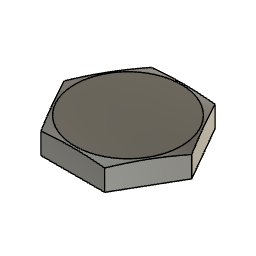
Main Wheel Holder (Autodesk Fusion 360 design; units mm, degrees)
Autodesk Fusion 360 part; units mm, degrees
sketch "Sketch1" plane through (0, 0, 0) normal (0, 0, 1) x (1, 0, 0) in component "Component"
  circle A0 centre (0, 0) radius 1.55
  circle A1 centre (0, 0) radius 2.75
  line L0 (-2.75, 0) -> (-1.375, -2.3816)
  line L1 (-1.375, -2.3816) -> (1.375, -2.3816)
  line L2 (1.375, -2.3816) -> (2.75, 0)
  line L3 (2.75, 0) -> (1.375, 2.3816)
  line L4 (1.375, 2.3816) -> (-1.375, 2.3816)
  line L5 (-1.375, 2.3816) -> (-2.75, 0)
  dimension "d1" = 3.1
  dimension "d2" = 5.5
  dimension "d12" = 4.7631
  constraint coincident A0.centre A1.centre
  constraint concentric A0 A1
  constraint coincident A1 L0.start
  measures "d1" diameter of A0
  measures "d2" diameter of A1
  measures "d12" distance of L0 L3
extrude "Extrude1" add sketch "Sketch1" along normal blind 1 contours A0 | L0 L1 L2 L3 L4 L5 in component "Component"
extrude "Extrude2" cut sketch "Sketch1" along normal blind 0.5 contours A0 in component "Component"
extrude "Extrude3" add 1 faces at (0.8338, -0.7144, 0.5) along direction (0, 0, -1) blind 0.2 in component "Component"
sketch "Sketch2" plane through (0, 0, 0) normal (0, 1, 0) x (1, 0, 0) in component "Component"
  line L0 (2.3, -1) -> (3.2799, -0.8006)
  line L1 (2.3, -1) -> (3.2799, -1) construction
  line L2 (3.2799, -0.8006) -> (3.2799, -1)
  line L3 (2.3, -1) -> (3.3, -1)
  dimension "d9" = 11.5
  dimension "d10" = 1
  constraint horizontal L1
  constraint perpendicular L1 L2
  measures "d9" angle of L0 L1
  measures "d10" distance of L0.start L0.end
revolve "Revolve1" cut sketch "Sketch2" angle 360 about axis through (0, 0, 1.75) along (0, 0, 1) in component "Component"
component "Component" placed x (1, 0, 0) y (0, 1, 0) z (0, 0, 1) at (0, 0, 0)
